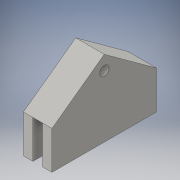
# Autodesk Inventor part: NarrowSupportForLift
Saved by Autodesk Inventor 2016 SP1 (Build 200210100, 210)
## iProperties
Created: 2016-02-14
Part Number: NarrowSupportForLift
Material: Generic
Document SubType Name: Modeling
Designer: steele
Density: 1 g/cm^3
Appearance: Default
Author: steele
Autodesk Inventor part; units mm, degrees
ref_plane "YZ Plane" through (0, 0, 0) normal (1, 0, 0) x (0, 1, 0)
ref_plane "XZ Plane" through (0, 0, 0) normal (0, 1, 0) x (-1, 0, 0)
ref_plane "XY Plane" through (0, 0, 0) normal (0, 0, 1) x (1, 0, 0)
sketch "Sketch4" plane through (0, 0, 0) normal (1, 0, 0) x (0, 1, 0)
  line L0 (-25.4, 34.925) -> (-25.4, -34.925)
  line L1 (-25.4, -34.925) -> (0, -34.925)
  line L2 (0, -34.925) -> (0, 34.925)
  line L3 (0, 34.925) -> (-25.4, 34.925)
  line L4 (-25.4, 34.925) -> (0, -34.925) construction
  line L5 (-25.4, -34.925) -> (0, 34.925) construction
  line L6 (0, 34.925) -> (25.4, 0)
  line L7 (25.4, 0) -> (0, -34.925)
  circle A0 centre (15.875, 0) radius 3.175
  point P0 (0, 0)
  point P1 (-12.7, 0)
  dimension "d1" = 12.7
  dimension "d2" = 69.85
  dimension "d3" = 25.4
  dimension "d4" = 6.35
  dimension "d10" = 25.4
  dimension "d11" = 9.525
  constraints: 16 end point, 2 midpoint, 2 parallel, 1 centre point, 1 equal length, 1 perpendicular, 1 vertical
  measures "d1" distance of point (0, 0) point (-12.7, 0)
  measures "d2" distance of L0.start L0.end
  measures "d3" distance of L2.end L0.start
  measures "d4" diameter of A0
  measures "d10" distance from line of L6.end L2
  measures "d11" distance of L6.end A0.centre
extrude "Extrusion1" add sketch "Sketch4" along normal mid plane 19.05
sketch "Sketch5" plane through (-9.525, -25.4, 34.925) normal (0, 0, 1) x (1, 0, 0)
  line L0 (0, 0) -> (19.05, 0) construction
  line L1 (9.525, 0) -> (9.525, 25.4) construction
  line L2 (6.35, 0) -> (12.7, 0)
  line L3 (12.7, 0) -> (12.7, 25.4)
  line L4 (12.7, 25.4) -> (6.35, 25.4)
  line L5 (6.35, 25.4) -> (6.35, 0)
  line L6 (6.35, 0) -> (12.7, 25.4) construction
  line L7 (12.7, 0) -> (6.35, 25.4) construction
  point P0 (9.525, 12.7)
  dimension "d7" = 6.35
  constraints: 14 end point, 4 midpoint, 2 parallel, 1 horizontal, 1 perpendicular, 1 vertical
  measures "d7" distance between parallel lines of L3 L5
extrude "Extrusion2" cut sketch "Sketch5" against normal through all
body "Solid1"
